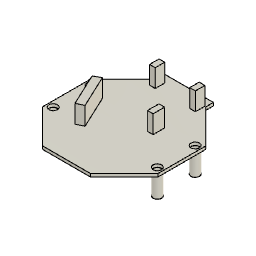
Board Enclosure (Autodesk Fusion 360 archive; units mm, degrees)
design "OpenBCI Cyton Board"
Autodesk Fusion 360 part; units mm, degrees
sketch "Sketch9" plane through (0, 0, 0) normal (0, 0, 1) x (1, 0, 0)
  line L0 (-30.5, -12.6335) -> (-12.6335, -30.5)
  line L1 (-12.6335, -30.5) -> (12.6335, -30.5)
  line L2 (12.6335, -30.5) -> (30.5, -12.6335)
  line L3 (30.5, -12.6335) -> (30.5, 12.6335)
  line L4 (30.5, 12.6335) -> (12.6335, 30.5)
  line L5 (12.6335, 30.5) -> (-12.6335, 30.5)
  line L6 (-12.6335, 30.5) -> (-30.5, 12.6335)
  line L7 (-30.5, 12.6335) -> (-30.5, -12.6335)
  line L8 (-12.6335, 30.5) -> (12.6335, 30.5)
  line L9 (12.6335, 30.5) -> (12.6335, 34.5)
  line L10 (12.6335, 34.5) -> (-12.6335, 34.5)
  line L11 (-12.6335, 34.5) -> (-12.6335, 30.5)
  dimension "d23" = 30.5
  dimension "d33" = 4
  constraint horizontal L8
  constraint vertical L9
  constraint horizontal L10
  constraint vertical L11
  measures "d23" distance of origin L7
  measures "d33" distance of L5.end L10.end
extrude "Extrude1" add sketch "Sketch9" along normal blind 1.6 makes body 1
sketch "Sketch11" plane through (0, 0, 1.6) normal (0, 0, 1) x (-1, 0, 0)
  line L0 (30.5, -12.6335) -> (30.5, 12.6335)
  line L1 (30.5, 12.6335) -> (12.6335, 30.5)
  line L2 (12.6335, 30.5) -> (-12.6335, 30.5)
  line L3 (-12.6335, 30.5) -> (-30.5, 12.6335)
  line L4 (-30.5, 12.6335) -> (-30.5, -12.6335)
  line L5 (-30.5, -12.6335) -> (-12.6335, -30.5)
  line L6 (12.6335, -30.5) -> (30.5, -12.6335)
  circle A0 centre (-27.5, -10) radius 2.25
  line L7 (0, 0) -> (0, -30.5) construction
  line L8 (0, 0) -> (30.5, 0) construction
  circle A1 centre (27.5, -10) radius 2.25
  circle A2 centre (27.5, 10) radius 2.25
  circle A3 centre (-27.5, 10) radius 2.25
  line L9 (12.6335, -34.5) -> (12.6335, -30.5)
  line L10 (-12.6335, -30.5) -> (-12.6335, -34.5)
  line L11 (-12.6335, -34.5) -> (12.6335, -34.5)
  dimension "d26" = 4.5
  dimension "d27" = 10
  dimension "d28" = 27.5
  constraint coincident L7.start L8.start
  constraint midpoint L0 L8.end
  constraint symmetric A0 L7 A1
  constraint symmetric A0 L8 A3
  constraint symmetric L8 A1 A2
  measures "d26" diameter of A0
  measures "d27" vertical distance of L7.start A0.centre
  measures "d28" horizontal distance of L7.start A0.centre
extrude "Extrude2" cut sketch "Sketch11" against normal through all contours A0 | A1 | A2 | A3 bodies 1
sketch "Sketch12" plane through (0, 0, 0) normal (0, 0, -1) x (1, 0, 0)
  circle A0 centre (-27.5, 10) radius 2.25
  circle A1 centre (27.5, 10) radius 2.25
  circle A2 centre (-27.5, -10) radius 2.25
  circle A3 centre (27.5, -10) radius 2.25
  line L0 (-30.5, 12.6335) -> (-30.5, -12.6335)
  line L1 (-30.5, -12.6335) -> (-12.6335, -30.5)
  line L2 (12.6335, -30.5) -> (30.5, -12.6335)
  line L3 (30.5, -12.6335) -> (30.5, 12.6335)
  line L4 (30.5, 12.6335) -> (12.6335, 30.5)
  line L5 (12.6335, 30.5) -> (-12.6335, 30.5)
  line L6 (-12.6335, 30.5) -> (-30.5, 12.6335)
  circle A4 centre (-27.5, 10) radius 2.25
  circle A5 centre (27.5, -10) radius 2.25
  circle A6 centre (27.5, -10) radius 2.1527
  line L7 (0, -30.5) -> (0, 30.5) construction
  line L8 (30.5, 0) -> (-30.5, 0) construction
  line L9 (27.5, -10) -> (0, -10) construction
  circle A7 centre (-27.5, -10) radius 2.1527
  circle A8 centre (-27.5, -10) radius 2.25
  line L10 (-27.5, -10) -> (0, -10) construction
  line L11 (27.5, -10) -> (27.5, 10) construction
  line L12 (-27.5, -10) -> (-27.5, 10) construction
  circle A9 centre (27.5, 10) radius 2.1527
  circle A10 centre (27.5, 10) radius 2.25
  circle A11 centre (-27.5, 10) radius 2.1527
  circle A12 centre (-27.5, 10) radius 2.25
  line L13 (27.5, 10) -> (27.5, -10) construction
  line L14 (-27.5, 10) -> (-27.5, -10) construction
  line L15 (-12.6335, -30.5) -> (-12.6335, -34.5)
  line L16 (-12.6335, -34.5) -> (12.6335, -34.5)
  line L17 (12.6335, -34.5) -> (12.6335, -30.5)
  constraint concentric A3 A5
  constraint concentric A5 A6
  constraint midpoint L5 L7.end
  constraint midpoint L3 L8.start
  constraint midpoint L0 L8.end
  constraint coincident A3.centre A5.centre
  constraint coincident L7 L9.end
  constraint perpendicular L7 L9
  constraint symmetric A5 L7 A8
  constraint symmetric A6 L7 A7
  constraint symmetric L7 A3.centre A2.centre
  constraint symmetric L7 L9.end L10.end
  constraint coincident A1.centre L11.end
  constraint coincident A2.centre A7.centre
  constraint coincident A0.centre A4.centre
  constraint perpendicular L10 L12
  constraint symmetric A5 L8 A10
  constraint symmetric A6 L8 A9
  constraint symmetric L8 A7 A11
  constraint symmetric L8 A8 A12
  constraint symmetric L8 A3.centre A1.centre
  constraint symmetric L8 A1.centre A3.centre
  constraint symmetric L8 A2.centre A0.centre
  constraint symmetric L8 A0.centre A2.centre
extrude "Extrude3" add sketch "Sketch12" along normal blind 11.43 separate body contours A0 A4 A12 | A1 A10 | A2 A8 | A3 A5 makes body 2 at (-25.2612, -9.776, -7.62) makes body 3 at (-25.2612, 10.224, -7.62) makes body 4 at (29.7388, -9.776, -7.62) makes body 5 at (29.7388, 10.224, -7.62)
sketch "Sketch13" plane through (0, 0, 1.6) normal (0, 0, 1) x (-1, 0, 0)
  circle A0 centre (27.5, 10) radius 2.25
  circle A1 centre (-27.5, 10) radius 2.25
  circle A2 centre (27.5, -10) radius 2.25
  circle A3 centre (-27.5, -10) radius 2.25
  line L0 (12.6335, -34.5) -> (12.6335, -30.5)
  line L1 (12.6335, -30.5) -> (30.5, -12.6335)
  line L2 (30.5, -12.6335) -> (30.5, 12.6335)
  line L3 (30.5, 12.6335) -> (12.6335, 30.5)
  line L4 (12.6335, 30.5) -> (-12.6335, 30.5)
  line L5 (-12.6335, 30.5) -> (-30.5, 12.6335)
  line L6 (-30.5, 12.6335) -> (-30.5, -12.6335)
  line L7 (-30.5, -12.6335) -> (-12.6335, -30.5)
  line L8 (-12.6335, -30.5) -> (-12.6335, -34.5)
  line L9 (-12.6335, -34.5) -> (12.6335, -34.5)
  line L10 (22, -5) -> (14, 12)
  line L11 (14, 12) -> (10.3858, 10.2992)
  line L12 (10.3858, 10.2992) -> (18.5347, -7.0172)
  line L13 (18.5347, -7.0172) -> (22, -5)
  line L14 (12.1173, -30.5) -> (9.1173, -30.5)
  line L15 (9.1173, -30.5) -> (9.1173, -25.5)
  line L16 (9.1173, -25.5) -> (12.1173, -25.5)
  line L17 (12.1173, -25.5) -> (12.1173, -30.5)
  line L18 (9.1173, -30.5) -> (0, -30.5) construction
  line L19 (0, -30.5) -> (0, -21.6781) construction
  line L20 (-12.1173, -30.5) -> (-9.1173, -30.5)
  line L21 (-9.1173, -30.5) -> (-9.1173, -25.5)
  line L22 (-12.1173, -25.5) -> (-12.1173, -30.5)
  line L23 (-9.1173, -25.5) -> (-12.1173, -25.5)
  line L24 (-9.1173, -30.5) -> (0, -30.5) construction
  line L25 (-11.4116, -35.3207) -> (-11.4116, -9.9207) construction
  line L26 (-11.4116, -9.9207) -> (-8.4116, -9.9207)
  line L27 (-8.4116, -9.9207) -> (-8.4116, -3.8247)
  line L28 (-8.4116, -3.8247) -> (-11.4116, -3.8247)
  line L29 (-11.4116, -3.8247) -> (-11.4116, -9.9207)
  dimension "d34" = 3
  dimension "d35" = 5
  dimension "d36" = 25.4
  dimension "d38" = 3
  dimension "d39" = 6.096
  constraint perpendicular L10 L11
  constraint perpendicular L11 L12
  constraint horizontal L14
  constraint vertical L15
  constraint horizontal L16
  constraint vertical L17
  constraint perpendicular L15 L18
  constraint perpendicular L9 L19
  constraint symmetric L14.start L19 L20.start
  constraint symmetric L14.end L19 L20.end
  constraint symmetric L15.end L19 L21.end
  constraint symmetric L16.end L19 L22.start
  constraint symmetric L18.end L19 L24.end
  constraint perpendicular L9 L25
  constraint horizontal L26
  constraint vertical L27
  constraint horizontal L28
  constraint vertical L29
  measures "d34" distance of L14.start L14.end
  measures "d35" distance of L14.start L16.end
  measures "d36" distance of L25.start L25.end
  measures "d38" distance of L25.end L26.end
  measures "d39" distance of L25.end L28.end
extrude "Extrude4" add sketch "Sketch13" along normal blind 9.525 contours L10 L11 L12 L13 | L14 L15 L16 L17 | L20 L21 L22 L23 | L26 L27 L28 L29 bodies 1
equation "d28 = ( 55 / 2 ) * 1 mm"
